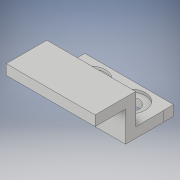
# Autodesk Inventor part: Pantalla - encaix slider
Saved by Autodesk Inventor 2019 (Build 230136000, 136)
## iProperties
Created: 2018-09-18
Part Number: Pantalla - encaix slider
Material: Genérico
Document SubType Name: Modeling
Designer: Albert Garangou Culebras
Density: 1 g/cm^3
Appearance: Valor por defecto
Author: Albert Garangou Culebras
Autodesk Inventor part; units mm, degrees
ref_plane "YZ Plane" through (0, 0, 0) normal (1, 0, 0) x (0, 1, 0)
ref_plane "XZ Plane" through (0, 0, 0) normal (0, 1, 0) x (-1, 0, 0)
ref_plane "XY Plane" through (0, 0, 0) normal (0, 0, 1) x (1, 0, 0)
sketch "Boceto1" plane through (0, 0, 0) normal (0, 1, 0) x (-1, 0, 0)
  line L0 (0, 0) -> (3.5, 0)
  line L1 (3.5, 0) -> (5.5, 0)
  line L2 (0, 0) -> (-2, 0)
  line L3 (-2, -5.5) -> (5.5, -5.5)
  line L4 (-2, 0) -> (-5, 0)
  line L5 (-5, -5.5) -> (-2, -5.5)
  line L6 (5.5, 0) -> (8.5, 0)
  line L7 (8.5, -5.5) -> (5.5, -5.5)
  line L8 (8.5, -5.5) -> (9.5, -5.5)
  line L9 (9.5, 0) -> (8.5, 0)
  line L10 (-5, -5.5) -> (-6, -5.5)
  line L11 (-6, 0) -> (-5, 0)
  line L12 (9.5, -5.5) -> (10.5, -5.5)
  line L13 (10.5, -5.5) -> (10.5, 0)
  line L14 (10.5, 0) -> (9.5, 0)
  line L15 (-6, -5.5) -> (-7, -5.5)
  line L16 (-7, -5.5) -> (-7, 0)
  line L17 (-7, 0) -> (-6, 0)
  dimension "d30" = 1
  dimension "d37" = 1
  dimension "d38" = 1
  constraints: 36 end point, 8 horizontal, 4 perpendicular, 1 collinear, 1 point on line
  measures "d30" distance of L5.start L10.end
  measures "d37" distance of L8.end L12.end
  measures "d38" distance of L10.end L15.end
extrude "Extrusión3" add sketch "Boceto1" along normal blind 2
sketch "Boceto4" plane through (-8.5, 0, 0) normal (0, 0, 1) x (1, 0, 0)
  line L0 (15.5, 2) -> (-2, 2) projected
  line L1 (0, 2) -> (13.5, 2)
  line L2 (13.5, 2) -> (13.5, 0)
  line L3 (13.5, 0) -> (0, 0)
  line L4 (0, 0) -> (0, 2)
  point P0 (8.5, 0)
  point P1 (14.5, 2)
  point P2 (-1, 2)
  constraints: 8 end point, 2 parallel, 1 horizontal, 1 perpendicular
extrude "Extrusión4" add sketch "Boceto4" along normal blind 2
sketch "Boceto5" plane through (0, 2, 0) normal (0, 1, 0) x (1, 0, 0)
  line L0 (-8.5, -2) -> (5, -2) projected
  line L1 (5, -2) -> (-8.5, -2)
  line L2 (-8.5, -2) -> (-8.5, 0)
  line L3 (-8.5, 0) -> (5, 0)
  line L4 (5, 0) -> (5, -2)
  point P0 (0, 0)
  constraints: 8 end point, 2 parallel, 1 horizontal, 1 perpendicular
extrude "Extrusión5" add sketch "Boceto5" along normal blind 6
sketch "Boceto6" plane through (-8.5, 0, 2) normal (0, 0, 1) x (1, 0, 0)
  line L0 (0, 0) -> (13.5, 0) projected
  line L1 (13.5, 0) -> (13.5, 6)
  line L2 (13.5, 6) -> (0, 6)
  line L3 (0, 0) -> (0, 6)
  line L4 (0, 0) -> (13.5, 0)
  line L5 (0, 0) -> (0, 8) projected
  line L6 (0, 8) -> (13.5, 8)
  line L7 (13.5, 8) -> (13.5, 6)
  line L8 (13.5, 6) -> (0, 6)
  line L9 (0, 6) -> (0, 8)
  point P0 (8.5, 0)
  constraints: 16 end point, 3 equal length, 3 perpendicular, 1 horizontal
extrude "Extrusión6" add sketch "Boceto6" along normal blind 5 contours L5 L6 L7 L2
sketch "Boceto8" plane through (5, 0, -5.5) normal (0, 0, -1) x (-1, 0, 0)
  line L0 (13.5, 0) -> (13.5, 6) projected
  line L1 (13.5, 2) -> (0, 2) projected
  line L2 (13.5, 0) -> (0, 0)
  line L3 (0, 0) -> (0, 2)
  line L4 (0, 2) -> (13.5, 2)
  line L5 (13.5, 2) -> (13.5, 0)
  point P0 (5, 0)
  constraints: 8 end point, 2 parallel, 1 horizontal, 1 perpendicular
extrude "Extrusión8" add sketch "Boceto8" along normal blind 2
sketch "Boceto11" plane through (5, 0, 2) normal (1, 0, 0) x (0, 0, -1)
  line L0 (-5, 8) -> (2, 8)
  line L1 (2, 8) -> (2, 6)
  line L2 (-5, 6) -> (-5, 8)
  line L3 (0, 0) -> (0, 6) projected
  line L4 (2, 0) -> (2, 2) projected
  line L5 (2, 6) -> (2, 0)
  line L6 (2, 0) -> (0, 0)
  line L7 (0, 0) -> (0, 6)
  line L8 (0, 6) -> (-5, 6) projected
  line L9 (0, 6) -> (-5, 6)
  line L10 (2, 0) -> (0, 0) projected
  line L11 (0, 0) -> (2, 0)
  line L12 (2, 2) -> (2, 8) projected
  line L13 (2, 0) -> (2, 8)
  line L14 (2, 8) -> (-5, 8) projected
  line L15 (2, 8) -> (-5, 8)
  line L16 (-5, 8) -> (-5, 6)
  line L17 (0, 6) -> (0, 0)
  constraints: 24 end point, 5 collinear, 2 horizontal, 2 parallel, 1 perpendicular
extrude "Extrusión11" add sketch "Boceto11" along normal blind 2
sketch "Boceto12" plane through (-8.5, 0, 0) normal (-1, 0, 0) x (0, 0, 1)
  line L0 (0, 8) -> (7, 8) projected
  line L1 (7, 8) -> (7, 6)
  line L2 (2, 6) -> (7, 6) projected
  line L3 (7, 6) -> (2, 6)
  line L4 (2, 6) -> (2, 0)
  line L5 (0, 0) -> (2, 0) projected
  line L6 (2, 0) -> (0, 0)
  line L7 (0, 2) -> (0, 8) projected
  line L8 (0, 0) -> (0, 8)
  line L9 (0, 8) -> (7, 8)
  constraints: 12 end point, 3 collinear, 1 parallel, 1 perpendicular, 1 vertical
extrude "Extrusión12" add sketch "Boceto12" along normal blind 2
sketch "Boceto13" plane through (0, 2, 0) normal (0, 1, 0) x (1, 0, 0)
  line L0 (-8.5, 5.5) -> (-10.5, 5.5) projected
  line L1 (-10.5, 5.5) -> (6.9708, 5.5)
  line L2 (6.9708, 5.5) -> (6.9708, 7.5)
  line L3 (6.9708, 7.5) -> (-10.5, 7.5)
  line L4 (-10.5, 7.5) -> (-10.5, 5.5)
  point P0 (0, 0)
  constraints: 8 end point, 2 parallel, 1 horizontal, 1 perpendicular
extrude "Extrusión13" add sketch "Boceto13" against normal blind 2
sketch "Boceto14" plane through (0, 2, 0) normal (0, 1, 0) x (1, 0, 0)
  circle A0 centre (2.1471, 3.7519) radius 1.75
  circle A1 centre (-5.6769, 3.7519) radius 1.75
  line L0 (1.1471, 3.7519) -> (2.1471, 3.7519)
  line L1 (-4.6769, 3.7519) -> (-5.6769, 3.7519)
  point P0 (0, 0)
  dimension "d43" = 3.5
  dimension "d44" = 3.5
  dimension "d45" = 1
  dimension "d46" = 1
  constraints: 4 end point, 2 centre point, 2 horizontal
  measures "d43" diameter of A0
  measures "d44" diameter of A1
  measures "d45" distance of L0.start L0.end
  measures "d46" distance of L1.start L1.end
extrude "Extrusión14" cut sketch "Boceto14" against normal blind 2
sketch "Boceto15" plane through (0, 2, 0) normal (0, 1, 0) x (1, 0, 0)
  circle A0 centre (2.1471, 3.7519) radius 1.75 projected
  circle A1 centre (2.1471, 3.7519) radius 3
  circle A2 centre (-5.6769, 3.7519) radius 1.75 projected
  circle A3 centre (-5.6769, 3.7519) radius 3
  point P0 (0, 0)
  dimension "d49" = 6
  dimension "d50" = 6
  constraints: 2 centre point, 2 coincident
  measures "d49" diameter of A1
  measures "d50" diameter of A3
extrude "Extrusión15" cut sketch "Boceto15" against normal blind 0.5
sketch "Boceto16" plane through (-8.5, 0, 7) normal (0, 0, 1) x (1, 0, 0)
  line L0 (15.5, 2) -> (15.5, 8) projected
  line L1 (15.5, 6) -> (-2, 6) projected
  line L2 (15.5, 8) -> (-2, 8)
  line L3 (-2, 8) -> (-2, 6)
  line L4 (-2, 6) -> (15.5, 6)
  line L5 (15.5, 6) -> (15.5, 8)
  point P0 (8.5, 0)
  constraints: 8 end point, 2 parallel, 1 horizontal, 1 perpendicular
extrude "Extrusión16" add sketch "Boceto16" along normal blind 1
